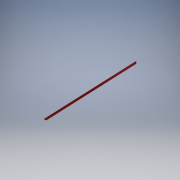
# Autodesk Inventor part: FE-00040-07_2_Red
Saved by Autodesk Inventor 2017.1 (Build 211199000, 199)
## iProperties
Created: 2017-01-05
Part Number: FE-00040-07_2_Red
Material: Generic
Document SubType Name: Modeling
Designer: PhillipD
Density: 1 g/cm^3
Appearance: Smooth - Red
Author: PhillipD
Autodesk Inventor part; units mm, degrees
ref_plane "YZ Plane" through (0, 0, 0) normal (1, 0, 0) x (0, 1, 0)
ref_plane "XZ Plane" through (0, 0, 0) normal (0, 1, 0) x (-1, 0, 0)
ref_plane "XY Plane" through (0, 0, 0) normal (0, 0, 1) x (1, 0, 0)
sketch "Sketch2" plane through (0, 0, 0) normal (0, 1, 0) x (-1, 0, 0)
  line L0 (0, 0) -> (2775.1802, -2898.9911)
  line L1 (2775.1802, -2898.9911) -> (2775.1802, -2825.529)
  line L2 (2775.1802, -2825.529) -> (70.3247, 0)
  line L3 (70.3247, 0) -> (0, 0)
  dimension "d12" = 50.8
  dimension "d13" = 136.25
  dimension "d14" = 4013.2
  constraints: 8 end point, 1 horizontal, 1 parallel, 1 vertical
  measures "d12" distance between parallel lines of L0 L2
  measures "d13" angle of L1 L2
  measures "d14" distance of L0.start L0.end
extrude "Extrusion3" add sketch "Sketch2" along normal blind 3.175
body "Solid3"
